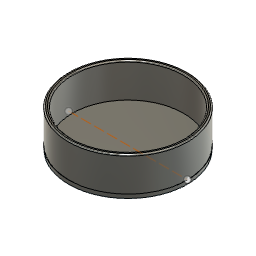
Bench block holder v1 (Autodesk Fusion 360 design; units mm, degrees)
Autodesk Fusion 360 part; units mm, degrees
sketch "Sketch1" plane through (0, 0, 0) normal (0, 1, 0) x (1, 0, 0)
  circle A0 centre (0, 0) radius 41.275
  dimension "d1" = 82.55
  constraint coincident A0.centre origin
  measures "d1" diameter of A0
extrude "Extrude1" add sketch "Sketch1" along normal blind 25.4 thin wall 3 outside makes body 1
sketch "Sketch2" plane through (0, 0, 0) normal (0, 1, 0) x (1, 0, 0)
  line L0 (-44, 0) -> (44, 0) construction
  dimension "d5" = 88
  constraint horizontal L0
  measures "d5" distance of L0.start L0.end
sketch "Sketch3" plane through (0, 0, 0) normal (0, 1, 0) x (1, 0, 0)
  circle A0 centre (0, 0) radius 44
  dimension "d6" = 88
  constraint coincident A0.centre origin
  measures "d6" diameter of A0
extrude "Extrude2" add sketch "Sketch3" against normal blind 3 bodies 1
sphere "SpherePrimitive1" add diameter 10 placed x (0, 0, -1) y (0, 1, 0) z (1, 0, 0) at (0, -26, 64) separate body makes body 2
move_body "MoveFace1" bodies 2 to x (1, 0, 0) y (0, 1, 0) z (0, 0, 1) at (17.459, 14.4885, -13.319) on bodies 2
move_body "MoveFace2" bodies 2 to x (1, 0, 0) y (0, 1, 0) z (0, 0, 1) at (-2.2314, -7.5198, -18.7842) on bodies 2
move_body "MoveFace3" bodies 2 to x (1, 0, 0) y (0, 1, 0) z (0, 0, 1) at (1.5233, 16.2898, -0.3957) on bodies 2
sketch "Sketch5" plane through (0, -3, 0) normal (0, -1, 0) x (1, 0, 0)
  circle A0 centre (0, 0) radius 44
sphere "SpherePrimitive2" add diameter 10 placed x (1, 0, 0) y (0, 0, -1) z (0, 1, 0) at (-65, 0, 15) separate body makes body 3
move_body "MoveFace4" bodies 3 to x (1, 0, 0) y (0, 1, 0) z (0, 0, 1) at (29.387, -5.6766, -12.7606) on bodies 3
move_body "MoveFace5" bodies 3 to x (1, 0, 0) y (0, 1, 0) z (0, 0, 1) at (-0.5266, 1.9809, -0.5696) on bodies 3
sphere "SpherePrimitive3" add diameter 10 placed x (1, 0, 0) y (0, 1, 0) z (0, 0, 1) at (-6, -15, 0) separate body makes body 4
move_body "MoveFace6" bodies 3 to x (1, 0, 0) y (0, 1, 0) z (0, 0, 1) at (-0.0682, 0.7511, -0.0314) on bodies 3
move_body "MoveFace7" bodies 4 to x (1, 0, 0) y (0, 1, 0) z (0, 0, 1) at (22.3357, -2.9357, -30.4189) on bodies 4
move_body "MoveFace8" bodies 4 to x (1, 0, 0) y (0, 1, 0) z (0, 0, 1) at (-1.5522, 14.9184, -0.4378) on bodies 4
move_body "MoveFace9" bodies 4 to x (1, 0, 0) y (0, 1, 0) z (0, 0, 1) at (2.4433, 1.2, -1.3066) on bodies 4
delete_face "DeleteFace1" 3 faces at (21.9671, -0.6354, -33.2273) (21.4913, -1.5596, 30.4373) (-31.4675, -1.7627, 0.5744) on bodies 2 3 4
fillet "Fillet1" radius 1 1 edges at (-38.4818, 25.4, -14.9257) on bodies 1
fillet "Fillet2" radius 1 1 edges at (-41.2788, 25.4, 16.0105) on bodies 1
